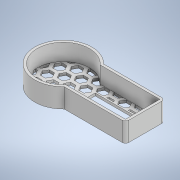
# Autodesk Inventor part: badge
Saved by Autodesk Inventor 2022 (Build 260153000, 153)
## iProperties
Created: 2019-12-22
Part Number: badge
Material: Generic
Document SubType Name: Modeling
Designer: user
Density: 1 g/cm^3
Appearance: Default
Author: user
## iProperties of the stored document _3DPrint.ipt
Created: 2019-12-23
Part Number: _3DPrint
Material: Generic
Document SubType Name: Modeling
Designer: user
Density: 1 g/cm^3
Appearance: Default
Author: user
Autodesk Inventor part; units mm, degrees
(part 1 of 2)
ref_plane "YZ Plane" through (0, 0, 0) normal (1, 0, 0) x (0, 1, 0)
ref_plane "XZ Plane" through (0, 0, 0) normal (0, 1, 0) x (-1, 0, 0)
ref_plane "XY Plane" through (0, 0, 0) normal (0, 0, 1) x (1, 0, 0)
sketch "Sketch1" plane through (0, 0, 0) normal (0, 1, 0) x (-1, 0, 0)
  line L0 (10.663939, 24.188791) -> (-74.736061, 24.188791)
  line L1 (-74.736061, -33.711209) -> (10.663939, -33.711209)
  line L2 (12.663939, 15.288573) -> (20.571727, 5.864438)
  line L3 (21.039638, 4.578863) -> (21.039638, -14.141384)
  line L4 (20.571727, -15.42696) -> (12.663939, -24.851094)
  circle A0 centre (-13.836061, -4.761209) radius 17
  line L5 (-62.621724, 4.988791) -> (-62.621724, -14.511209)
  line L6 (-60.621724, -16.511209) -> (-26.121724, -16.511209)
  line L7 (-26.121724, 6.988791) -> (-60.621724, 6.988791)
  arc A1 (-62.621724, -14.511209) -> (-60.621724, -16.511209) centre (-60.621724, -14.511209) ccw
  arc A2 (-60.621724, 6.988791) -> (-62.621724, 4.988791) centre (-60.621724, 4.988791) ccw
  line L8 (-28.586061, -0.511209) -> (-55.121724, -0.511209)
  line L9 (-55.121724, -0.511209) -> (-55.121724, -9.011209)
  line L10 (-55.121724, -9.011209) -> (-28.586061, -9.011209)
  line L11 (-28.586061, -9.011209) -> (-28.586061, -0.511209)
  line L12 (-76.736061, 6.188791) -> (-76.736061, 22.188791)
  line L13 (-76.736061, -15.711209) -> (-76.736061, -31.711209)
  line L14 (9.163939, 22.688791) -> (-73.236061, 22.688791)
  line L15 (-73.236061, -32.211209) -> (9.163939, -32.211209)
  line L16 (11.163939, -30.211209) -> (11.163939, 20.688791)
  line L17 (-75.236061, 20.688791) -> (-75.236061, 4.86332)
  line L18 (-75.236061, -30.211209) -> (-75.236061, -14.385738)
  line L19 (12.663939, 22.188791) -> (12.663939, 15.288573)
  line L20 (12.663939, -24.851094) -> (12.663939, -31.711209)
  arc A3 (-76.736061, -31.711209) -> (-74.736061, -33.711209) centre (-74.736061, -31.711209) ccw
  arc A4 (-75.236061, -30.211209) -> (-73.236061, -32.211209) centre (-73.236061, -30.211209) ccw
  arc A5 (-73.236061, 22.688791) -> (-75.236061, 20.688791) centre (-73.236061, 20.688791) ccw
  arc A6 (-74.736061, 24.188791) -> (-76.736061, 22.188791) centre (-74.736061, 22.188791) ccw
  arc A7 (12.663939, 22.188791) -> (10.663939, 24.188791) centre (10.663939, 22.188791) ccw
  arc A8 (11.163939, 20.688791) -> (9.163939, 22.688791) centre (9.163939, 20.688791) ccw
  arc A9 (9.163939, -32.211209) -> (11.163939, -30.211209) centre (9.163939, -30.211209) ccw
  arc A10 (10.663939, -33.711209) -> (12.663939, -31.711209) centre (10.663939, -31.711209) ccw
  arc A11 (20.571727, -15.42696) -> (21.039638, -14.141384) centre (19.039638, -14.141384) ccw
  arc A12 (21.039638, 4.578863) -> (20.571727, 5.864438) centre (19.039638, 4.578863) ccw
  arc A13 (-76.736061, -15.711209) -> (-76.736061, 6.188791) centre (-85.076375, -4.761209) ccw
  circle A14 centre (16.664118, 5.166112) radius 1.75
  circle A15 centre (16.664118, -14.728633) radius 1.75
  line L21 (12.663939, 15.288573) -> (12.663939, -24.851094)
  line L22 (18.425716, 0.463151) -> (18.425716, -9.93338)
  line L23 (14.925716, 0.440313) -> (14.925716, -10.09463)
  arc A16 (14.925716, -10.09463) -> (18.425716, -9.93338) centre (16.664118, -9.762269) ccw
  arc A17 (18.425716, 0.463151) -> (14.925716, 0.440313) centre (16.67736, 0.199747) ccw
  point P0 (0, 0)
  point P1 (12.663939, 24.188791)
  point P2 (-76.736061, -33.711209)
  point P3 (-76.736061, 24.188791)
  point P4 (12.663939, -33.711209)
  point P5 (21.039638, -14.869325)
  point P6 (-62.621724, -16.511209)
  dimension "d19" = 18
  dimension "d20" = 34
  dimension "d26" = 2
  dimension "d28" = 7.5
  dimension "d32" = 7.5
  dimension "d33" = 7.5
  dimension "d36" = 1.5
  dimension "d37" = 1.5
  dimension "d40" = 1.5
  dimension "d41" = 2
  dimension "d84" = 54.9
  dimension "d89" = 18
  dimension "d104" = 86.4
  dimension "d110" = 13.76457
  dimension "d116" = 1.5
  dimension "d122" = 3.5
  dimension "d123" = 3.5
  dimension "d124" = 3.44228
  dimension "d125" = 3.44228
  dimension "d155" = 25
  dimension "d163" = 15.7
  dimension "d164" = 15.7
  dimension "d165" = 27.45
  dimension "d166" = 27.45
  dimension "d167" = 8.5
  dimension "d171" = 26.53566
  dimension "d173" = 39.75
  dimension "d213" = 4.00018
  dimension "d214" = 4.00018
  dimension "d219" = 140
  dimension "d221" = 140
  dimension "d246" = 4.96636
  dimension "d247" = 4.96636
  dimension "d248" = 13.5
  dimension "d249" = 1.5
  dimension "d250" = 1.5
  dimension "d251" = 4.00018
  dimension "d262" = 3.5
  dimension "d263" = 2.61392
  constraints: 48 end point, 34 point on circle, 24 tangent, 18 centre point, 13 point on line, 10 equal radius, 6 vertical, 5 parallel, 3 horizontal, 3 perpendicular, 2 collinear
  measures "d19" distance of point (-76.736, 24.189) L12.start
  measures "d20" diameter of A0
  measures "d26" radius of A1
  measures "d28" distance between parallel lines of L6 L10
  measures "d32" distance between parallel lines of L8 L7
  measures "d33" distance between parallel lines of L5 L9
  measures "d36" distance between parallel lines of L0 L14
  measures "d37" distance between parallel lines of L1 L15
  measures "d40" distance between parallel lines of L13 L18
  measures "d41" radius of A3
  measures "d84" distance between parallel lines of L15 L14
  measures "d89" distance of L13.start point (-76.736, -33.711)
  measures "d104" distance between parallel lines of L17 L16
  measures "d110" radius of A13
  measures "d116" distance between parallel lines of L17 L12
  measures "d122" diameter of A15
  measures "d123" diameter of A14
  measures "d124" distance from line of L4 A15.centre
  measures "d125" distance from line of L2 A14.centre
  measures "d155" distance from line of L16 A0.centre
  measures "d163" distance between parallel lines of L15 L6
  measures "d164" distance between parallel lines of L14 L7
  measures "d165" distance from line of L15 A0.centre
  measures "d166" distance from line of L14 A0.centre
  measures "d167" distance between parallel lines of L8 L10
  measures "d171" distance between parallel lines of L9 L11
  measures "d173" distance between parallel lines of L16 L11
  measures "d213" distance from line of L21 A14.centre
  measures "d214" distance from line of L21 A15.centre
  measures "d219" angle of L19 L2
  measures "d221" angle of L20 L4
  measures "d246" distance of A17.centre A14.centre
  measures "d247" distance of A15.centre A16.centre
  measures "d249" distance between parallel lines of L16 L19
  measures "d250" distance between parallel lines of L16 L20
  measures "d251" distance from line of L21 A16.centre
  measures "d262" distance between parallel lines of L23 L22
  measures "d263" distance from line of L3 L22.end
sketch "Sketch1 outline for TokenBuffer" plane through (0, 0, 0) normal (0, 1, 0) x (-1, 0, 0)
  line L0 (-26.121724, 6.988791) -> (-60.621724, 6.988791)
  arc A0 (-26.121724, -16.511209) -> (-26.121724, 6.988791) centre (-13.836061, -4.761209) ccw
  arc A1 (-60.621724, 6.988791) -> (-62.621724, 4.988791) centre (-60.621724, 4.988791) ccw
  line L1 (-60.621724, -16.511209) -> (-26.121724, -16.511209)
  line L2 (-62.621724, 4.988791) -> (-62.621724, -14.511209)
  arc A2 (-62.621724, -14.511209) -> (-60.621724, -16.511209) centre (-60.621724, -14.511209) ccw
  line L3 (-55.121724, -0.511209) -> (-28.586061, -0.511209)
  line L4 (-55.121724, -9.011209) -> (-55.121724, -0.511209)
  line L5 (-28.586061, -9.011209) -> (-55.121724, -9.011209)
  line L6 (-28.586061, -0.511209) -> (-28.586061, -9.011209)
extrude "TokenBuffer" add sketch "Sketch1 outline for TokenBuffer" against normal blind 10
sketch "Sketch4" plane through (0, 0, 0) normal (0, 1, 0) x (1, 0, 0)
  arc A0 (26.121724, 16.511209) -> (26.121724, -6.988791) centre (13.836061, 4.761209) ccw
  circle A1 centre (13.836061, 4.761209) radius 15.5
  line L0 (25.463077, -5.488791) -> (61.121724, -5.488791)
  line L1 (61.121724, -5.488791) -> (61.121724, 15.011209)
  line L2 (61.121724, 15.011209) -> (25.463077, 15.011209)
  line L3 (25.463077, 15.011209) -> (25.463077, -5.488791)
  line L4 (60.621724, -6.988791) -> (26.121724, -6.988791)
  line L5 (26.121724, 16.511209) -> (60.621724, 16.511209)
  line L6 (62.621724, 14.511209) -> (62.621724, -4.988791)
  point P0 (0, 0)
  point P1 (25.463077, 15.011209)
  point P2 (25.463077, 15.011209)
  dimension "d56" = 1.5
  dimension "d57" = 1.5
  dimension "d58" = 1.5
  dimension "d59" = 1.5
  constraints: 8 end point, 2 parallel, 1 coincident, 1 horizontal, 1 perpendicular, 3 other
  measures "d57" distance between parallel lines of L4 L0
  measures "d58" distance between parallel lines of L5 L2
  measures "d59" distance between parallel lines of L6 L1
sketch "Sketch4 outline for TokenCut" plane through (0, 0, 0) normal (0, 1, 0) x (1, 0, 0)
  arc A0 (25.463077, 15.011209) -> (25.463077, -5.488791) centre (13.836061, 4.761209) ccw
  line L0 (61.121724, 15.011209) -> (25.463077, 15.011209)
  line L1 (61.121724, -5.488791) -> (61.121724, 15.011209)
  line L2 (25.463077, -5.488791) -> (61.121724, -5.488791)
extrude "TokenCut" cut sketch "Sketch4 outline for TokenCut" against normal blind 8.5
sketch "Sketch12" plane through (0, 0, 0) normal (0, 1, 0) x (1, 0, 0)
  arc A0 (25.463077, 15.011209) -> (25.463077, -5.488791) centre (13.836061, 4.761209) ccw
  circle A1 centre (13.836061, 4.761209) radius 15.5
  line L0 (60.621724, -6.988791) -> (26.121724, -6.988791)
  line L1 (26.121724, -6.988791) -> (60.621724, -6.988791)
  line L2 (62.621724, 14.511209) -> (62.621724, -4.988791)
  arc A2 (60.621724, -6.988791) -> (62.621724, -4.988791) centre (60.621724, -4.988791) ccw
  line L3 (61.121724, -5.488791) -> (25.463077, -5.488791)
  line L4 (25.463077, -5.488791) -> (61.121724, -5.488791)
  line L5 (61.121724, 15.011209) -> (61.121724, -5.488791)
  line L6 (61.121724, -5.488791) -> (61.121724, 15.011209)
  line L7 (25.463077, 15.011209) -> (61.121724, 15.011209)
  line L8 (61.121724, 15.011209) -> (25.463077, 15.011209)
  line L9 (62.621724, -4.988791) -> (63.064996, 19.511209)
  line L10 (62.621724, 14.511209) -> (62.621724, -4.988791)
  line L11 (62.621724, -4.988791) -> (62.621724, 14.511209)
  line L12 (26.121724, 16.511209) -> (60.621724, 16.511209)
  arc A3 (62.621724, 14.511209) -> (60.621724, 16.511209) centre (60.621724, 14.511209) ccw
  line L13 (60.621724, 16.511209) -> (26.121724, 16.511209)
  circle A4 centre (13.836061, 4.761209) radius 17
  point P0 (0, 0)
  point P1 (26.121724, 16.511209)
  dimension "d152" = 34
  constraints: 14 end point, 4 centre point, 4 point on circle, 2 coincident, 2 horizontal, 2 perpendicular, 1 collinear, 1 tangent
  measures "d152" diameter of A4
sketch "Sketch12 outline for TokenAddition" plane through (0, 0, 0) normal (0, 1, 0) x (1, 0, 0)
  arc A0 (26.121724, 16.511209) -> (26.121724, -6.988791) centre (13.836061, 4.761209) ccw
  line L0 (60.621724, 16.511209) -> (26.121724, 16.511209)
  line L1 (26.121724, -6.988791) -> (60.621724, -6.988791)
  arc A1 (62.621724, 14.511209) -> (60.621724, 16.511209) centre (60.621724, 14.511209) ccw
  arc A2 (60.621724, -6.988791) -> (62.621724, -4.988791) centre (60.621724, -4.988791) ccw
  line L2 (62.621724, -4.988791) -> (62.621724, 14.511209)
  line L3 (25.463077, 15.011209) -> (61.121724, 15.011209)
  arc A3 (25.463077, -5.488791) -> (25.463077, 15.011209) centre (13.836061, 4.761209) cw
  line L4 (61.121724, -5.488791) -> (25.463077, -5.488791)
  line L5 (61.121724, 15.011209) -> (61.121724, -5.488791)
extrude "TokenAddition" add sketch "Sketch12 outline for TokenAddition" along normal blind 1.5
sketch "Sketch23" plane through (0, -10, 0) normal (0, -1, 0) x (1, 0, 0)
  line L0 (7.80058, -8.259557) -> (9.35908, -5.560156)
  line L1 (9.35908, -5.560156) -> (12.47608, -5.560156)
  line L2 (12.47608, -5.560156) -> (14.03458, -8.259557)
  line L3 (14.03458, -8.259557) -> (12.47608, -10.958958)
  line L4 (12.47608, -10.958958) -> (9.35908, -10.958958)
  line L5 (9.35908, -10.958958) -> (7.80058, -8.259557)
  line L6 (6.645879, -8.259557) -> (8.781729, -4.560156)
  line L7 (8.781729, -4.560156) -> (13.05343, -4.560156)
  line L8 (13.05343, -4.560156) -> (15.18928, -8.259557)
  line L9 (15.18928, -8.259557) -> (13.05343, -11.958958)
  line L10 (13.05343, -11.958958) -> (8.781729, -11.958958)
  line L11 (8.781729, -11.958958) -> (6.645879, -8.259557)
  line L12 (18.883631, -1.860755) -> (15.766631, -1.860755)
  line L13 (15.766631, -1.860755) -> (14.208131, -4.560156)
  line L14 (14.208131, -4.560156) -> (15.766631, -7.259557)
  line L15 (15.766631, -7.259557) -> (18.883631, -7.259557)
  line L16 (18.883631, -7.259557) -> (20.442131, -4.560156)
  line L17 (20.442131, -4.560156) -> (18.883631, -1.860755)
  line L18 (19.460981, -0.860755) -> (15.18928, -0.860755)
  line L19 (15.18928, -0.860755) -> (13.05343, -4.560156)
  line L20 (15.18928, -8.259557) -> (19.460981, -8.259557)
  line L21 (19.460981, -8.259557) -> (21.596831, -4.560156)
  line L22 (21.596831, -4.560156) -> (19.460981, -0.860755)
  line L23 (31.698732, 5.538047) -> (28.581732, 5.538047)
  line L24 (28.581732, 5.538047) -> (27.023232, 2.838646)
  line L25 (27.023232, 2.838646) -> (28.581732, 0.139245)
  line L26 (28.581732, 0.139245) -> (31.698732, 0.139245)
  line L27 (31.698732, 0.139245) -> (33.257232, 2.838646)
  line L28 (33.257232, 2.838646) -> (31.698732, 5.538047)
  line L29 (32.276082, 6.538047) -> (28.004382, 6.538047)
  line L30 (28.004382, 6.538047) -> (25.868532, 2.838646)
  line L31 (25.868532, 2.838646) -> (28.004382, -0.860755)
  line L32 (28.004382, -0.860755) -> (32.276082, -0.860755)
  line L33 (32.276082, -0.860755) -> (34.411933, 2.838646)
  line L34 (34.411933, 2.838646) -> (32.276082, 6.538047)
  line L35 (20.615681, -0.860755) -> (22.174181, 1.838646)
  line L36 (22.174181, 1.838646) -> (25.291181, 1.838646)
  line L37 (25.291181, 1.838646) -> (26.849681, -0.860755)
  line L38 (26.849681, -0.860755) -> (25.291181, -3.560156)
  line L39 (25.291181, -3.560156) -> (22.174181, -3.560156)
  line L40 (22.174181, -3.560156) -> (20.615681, -0.860755)
  line L41 (19.460981, -0.860755) -> (21.596831, 2.838646)
  line L42 (21.596831, 2.838646) -> (25.868532, 2.838646)
  line L43 (28.004382, -0.860755) -> (25.868532, -4.560156)
  line L44 (25.868532, -4.560156) -> (21.596831, -4.560156)
  line L45 (7.80058, -0.860755) -> (9.35908, -3.560156)
  line L46 (9.35908, -3.560156) -> (12.47608, -3.560156)
  line L47 (12.47608, -3.560156) -> (14.03458, -0.860755)
  line L48 (14.03458, -0.860755) -> (12.47608, 1.838646)
  line L49 (12.47608, 1.838646) -> (9.35908, 1.838646)
  line L50 (9.35908, 1.838646) -> (7.80058, -0.860755)
  line L51 (6.645879, -0.860755) -> (8.781729, -4.560156)
  line L52 (13.05343, -4.560156) -> (15.18928, -0.860755)
  line L53 (15.18928, -0.860755) -> (13.05343, 2.838646)
  line L54 (13.05343, 2.838646) -> (8.781729, 2.838646)
  line L55 (8.781729, 2.838646) -> (6.645879, -0.860755)
  line L56 (8.781729, 10.237449) -> (13.05343, 10.237449)
  line L57 (15.18928, 6.538047) -> (13.05343, 10.237449)
  line L58 (7.80058, 6.538047) -> (9.35908, 9.237449)
  line L59 (9.35908, 9.237449) -> (12.47608, 9.237449)
  line L60 (12.47608, 3.838646) -> (9.35908, 3.838646)
  line L61 (9.35908, 3.838646) -> (7.80058, 6.538047)
  line L62 (6.645879, 6.538047) -> (8.781729, 10.237449)
  line L63 (8.781729, 2.838646) -> (6.645879, 6.538047)
  line L64 (12.47608, 9.237449) -> (14.03458, 6.538047)
  line L65 (15.18928, 6.538047) -> (13.05343, 2.838646)
  line L66 (14.03458, 6.538047) -> (12.47608, 3.838646)
  line L67 (6.645879, -0.860755) -> (8.781729, 2.838646)
  line L68 (6.645879, 6.538047) -> (2.374179, 6.538047)
  line L69 (6.068529, 5.538047) -> (2.951529, 5.538047)
  line L70 (2.951529, 5.538047) -> (1.393029, 2.838646)
  line L71 (2.374179, 6.538047) -> (0.238328, 2.838646)
  line L72 (2.374179, -0.860755) -> (0.238328, 2.838646)
  line L73 (1.393029, 2.838646) -> (2.951529, 0.139245)
  line L74 (2.951529, 0.139245) -> (6.068529, 0.139245)
  line L75 (2.374179, -0.860755) -> (6.645879, -0.860755)
  line L76 (6.068529, 0.139245) -> (7.627029, 2.838646)
  line L77 (7.627029, 2.838646) -> (6.068529, 5.538047)
  line L78 (8.781729, -4.560156) -> (6.645879, -0.860755)
  line L79 (8.781729, -4.560156) -> (6.645879, -8.259557)
  line L80 (1.393029, -4.560156) -> (2.951529, -1.860755)
  line L81 (2.374179, -0.860755) -> (0.238328, -4.560156)
  line L82 (2.374179, -8.259557) -> (0.238328, -4.560156)
  line L83 (6.068529, -7.259557) -> (2.951529, -7.259557)
  line L84 (6.645879, -8.259557) -> (2.374179, -8.259557)
  line L85 (2.951529, -7.259557) -> (1.393029, -4.560156)
  line L86 (6.068529, -1.860755) -> (7.627029, -4.560156)
  line L87 (2.951529, -1.860755) -> (6.068529, -1.860755)
  line L88 (7.627029, -4.560156) -> (6.068529, -7.259557)
  line L89 (6.645879, -8.259557) -> (8.781729, -11.958958)
  line L90 (6.645879, -15.65836) -> (8.781729, -11.958958)
  line L91 (2.374179, -15.65836) -> (6.645879, -15.65836)
  line L92 (2.951529, -14.65836) -> (6.068529, -14.65836)
  line L93 (6.068529, -14.65836) -> (7.627029, -11.958958)
  line L94 (7.627029, -11.958958) -> (6.068529, -9.259557)
  line L95 (6.068529, -9.259557) -> (2.951529, -9.259557)
  line L96 (2.374179, -8.259557) -> (0.238328, -11.958958)
  line L97 (2.951529, -9.259557) -> (1.393029, -11.958958)
  line L98 (1.393029, -11.958958) -> (2.951529, -14.65836)
  line L99 (2.374179, -15.65836) -> (0.238328, -11.958958)
  line L100 (8.781729, -11.958958) -> (13.05343, -11.958958)
  line L101 (13.05343, -11.958958) -> (15.18928, -15.65836)
  line L102 (9.35908, -18.357761) -> (7.80058, -15.65836)
  line L103 (8.781729, -19.357761) -> (6.645879, -15.65836)
  line L104 (7.80058, -15.65836) -> (9.35908, -12.958958)
  line L105 (9.35908, -12.958958) -> (12.47608, -12.958958)
  line L106 (12.47608, -12.958958) -> (14.03458, -15.65836)
  line L107 (14.03458, -15.65836) -> (12.47608, -18.357761)
  line L108 (15.18928, -15.65836) -> (13.05343, -19.357761)
  line L109 (12.47608, -18.357761) -> (9.35908, -18.357761)
  line L110 (8.781729, -19.357761) -> (13.05343, -19.357761)
  line L111 (21.596831, 2.838646) -> (19.460981, -0.860755)
  line L112 (15.18928, -0.860755) -> (19.460981, -0.860755)
  line L113 (18.883631, 5.538047) -> (20.442131, 2.838646)
  line L114 (20.442131, 2.838646) -> (18.883631, 0.139245)
  line L115 (14.208131, 2.838646) -> (15.766631, 5.538047)
  line L116 (15.766631, 5.538047) -> (18.883631, 5.538047)
  line L117 (19.460981, 6.538047) -> (21.596831, 2.838646)
  line L118 (13.05343, 2.838646) -> (15.18928, 6.538047)
  line L119 (15.18928, 6.538047) -> (19.460981, 6.538047)
  line L120 (18.883631, 0.139245) -> (15.766631, 0.139245)
  line L121 (15.766631, 0.139245) -> (14.208131, 2.838646)
  line L122 (19.460981, -8.259557) -> (15.18928, -8.259557)
  line L123 (18.883631, -9.259557) -> (15.766631, -9.259557)
  line L124 (15.18928, -8.259557) -> (13.05343, -11.958958)
  line L125 (15.766631, -9.259557) -> (14.208131, -11.958958)
  line L126 (14.208131, -11.958958) -> (15.766631, -14.65836)
  line L127 (15.766631, -14.65836) -> (18.883631, -14.65836)
  line L128 (15.18928, -15.65836) -> (19.460981, -15.65836)
  line L129 (18.883631, -14.65836) -> (20.442131, -11.958958)
  line L130 (21.596831, -11.958958) -> (19.460981, -15.65836)
  line L131 (20.442131, -11.958958) -> (18.883631, -9.259557)
  line L132 (21.596831, -11.958958) -> (19.460981, -8.259557)
  line L133 (21.596831, -4.560156) -> (25.868532, -4.560156)
  line L134 (21.596831, -4.560156) -> (19.460981, -8.259557)
  line L135 (25.868532, -4.560156) -> (28.004382, -8.259557)
  line L136 (25.291181, -5.560156) -> (26.849681, -8.259557)
  line L137 (22.174181, -5.560156) -> (25.291181, -5.560156)
  line L138 (22.174181, -10.958958) -> (20.615681, -8.259557)
  line L139 (20.615681, -8.259557) -> (22.174181, -5.560156)
  line L140 (25.291181, -10.958958) -> (22.174181, -10.958958)
  line L141 (21.596831, -11.958958) -> (25.868532, -11.958958)
  line L142 (28.004382, -8.259557) -> (25.868532, -11.958958)
  line L143 (26.849681, -8.259557) -> (25.291181, -10.958958)
  line L144 (33.430783, 6.538047) -> (34.989283, 9.237449)
  line L145 (34.989283, 9.237449) -> (38.106283, 9.237449)
  line L146 (38.106283, 9.237449) -> (39.664783, 6.538047)
  line L147 (39.664783, 6.538047) -> (38.106283, 3.838646)
  line L148 (38.106283, 3.838646) -> (34.989283, 3.838646)
  line L149 (34.989283, 3.838646) -> (33.430783, 6.538047)
  line L150 (38.683633, 10.237449) -> (40.819483, 6.538047)
  line L151 (40.819483, 6.538047) -> (38.683633, 2.838646)
  line L152 (34.411933, 10.237449) -> (38.683633, 10.237449)
  line L153 (38.683633, 2.838646) -> (34.411933, 2.838646)
  line L154 (32.276082, 6.538047) -> (34.411933, 10.237449)
  line L155 (25.868532, 2.838646) -> (28.004382, 6.538047)
  line L156 (25.868532, 2.838646) -> (21.596831, 2.838646)
  line L157 (28.004382, 6.538047) -> (25.868532, 10.237449)
  line L158 (21.596831, 10.237449) -> (25.868532, 10.237449)
  line L159 (26.849681, 6.538047) -> (25.291181, 9.237449)
  line L160 (25.291181, 9.237449) -> (22.174181, 9.237449)
  line L161 (21.596831, 10.237449) -> (19.460981, 6.538047)
  line L162 (22.174181, 9.237449) -> (20.615681, 6.538047)
  line L163 (20.615681, 6.538047) -> (22.174181, 3.838646)
  line L164 (22.174181, 3.838646) -> (25.291181, 3.838646)
  line L165 (25.291181, 3.838646) -> (26.849681, 6.538047)
  line L166 (19.460981, 13.93685) -> (15.18928, 13.93685)
  line L167 (19.460981, 13.93685) -> (21.596831, 10.237449)
  line L168 (15.18928, 13.93685) -> (13.05343, 10.237449)
  line L169 (15.18928, 6.538047) -> (13.05343, 10.237449)
  line L170 (15.766631, 12.93685) -> (14.208131, 10.237449)
  line L171 (14.208131, 10.237449) -> (15.766631, 7.538047)
  line L172 (15.766631, 7.538047) -> (18.883631, 7.538047)
  line L173 (18.883631, 7.538047) -> (20.442131, 10.237449)
  line L174 (19.460981, 6.538047) -> (21.596831, 10.237449)
  line L175 (20.442131, 10.237449) -> (18.883631, 12.93685)
  line L176 (18.883631, 12.93685) -> (15.766631, 12.93685)
  line L177 (13.05343, 17.636251) -> (8.781729, 17.636251)
  line L178 (6.645879, 13.93685) -> (8.781729, 10.237449)
  line L179 (7.80058, 13.93685) -> (9.35908, 11.237449)
  line L180 (9.35908, 11.237449) -> (12.47608, 11.237449)
  line L181 (15.18928, 13.93685) -> (13.05343, 10.237449)
  line L182 (12.47608, 11.237449) -> (14.03458, 13.93685)
  line L183 (14.03458, 13.93685) -> (12.47608, 16.636251)
  line L184 (15.18928, 13.93685) -> (13.05343, 17.636251)
  line L185 (12.47608, 16.636251) -> (9.35908, 16.636251)
  line L186 (8.781729, 17.636251) -> (6.645879, 13.93685)
  line L187 (9.35908, 16.636251) -> (7.80058, 13.93685)
  line L188 (8.781729, 10.237449) -> (6.645879, 13.93685)
  line L189 (8.781729, 10.237449) -> (6.645879, 6.538047)
  line L190 (1.393029, 10.237449) -> (2.951529, 12.93685)
  line L191 (2.374179, 13.93685) -> (0.238328, 10.237449)
  line L192 (2.374179, 6.538047) -> (0.238328, 10.237449)
  line L193 (6.068529, 7.538047) -> (2.951529, 7.538047)
  line L194 (2.951529, 7.538047) -> (1.393029, 10.237449)
  line L195 (6.068529, 12.93685) -> (7.627029, 10.237449)
  line L196 (2.951529, 12.93685) -> (6.068529, 12.93685)
  line L197 (2.374179, 13.93685) -> (6.645879, 13.93685)
  line L198 (7.627029, 10.237449) -> (6.068529, 7.538047)
  line L199 (-6.169222, -0.860755) -> (-4.033372, 2.838646)
  line L200 (0.238328, 2.838646) -> (-4.033372, 2.838646)
  line L201 (2.374179, -0.860755) -> (0.238328, 2.838646)
  line L202 (1.219478, -0.860755) -> (-0.339022, 1.838646)
  line L203 (-0.339022, 1.838646) -> (-3.456022, 1.838646)
  line L204 (-3.456022, 1.838646) -> (-5.014522, -0.860755)
  line L205 (-6.169222, -0.860755) -> (-4.033372, -4.560156)
  line L206 (-5.014522, -0.860755) -> (-3.456022, -3.560156)
  line L207 (-4.033372, -4.560156) -> (0.238328, -4.560156)
  line L208 (-3.456022, -3.560156) -> (-0.339022, -3.560156)
  line L209 (-0.339022, -3.560156) -> (1.219478, -0.860755)
  line L210 (-4.033372, -4.560156) -> (0.238328, -4.560156)
  line L211 (0.238328, -4.560156) -> (2.374179, -8.259557)
  line L212 (-3.456022, -10.958958) -> (-5.014522, -8.259557)
  line L213 (-4.033372, -11.958958) -> (-6.169222, -8.259557)
  line L214 (-5.014522, -8.259557) -> (-3.456022, -5.560156)
  line L215 (-6.169222, -8.259557) -> (-4.033372, -4.560156)
  line L216 (-3.456022, -5.560156) -> (-0.339022, -5.560156)
  line L217 (-0.339022, -5.560156) -> (1.219478, -8.259557)
  line L218 (1.219478, -8.259557) -> (-0.339022, -10.958958)
  line L219 (-0.339022, -10.958958) -> (-3.456022, -10.958958)
  line L220 (-4.033372, -11.958958) -> (0.238328, -11.958958)
  line L221 (19.460981, -15.65836) -> (21.596831, -19.357761)
  line L222 (19.460981, -23.057162) -> (21.596831, -19.357761)
  line L223 (18.883631, -22.057162) -> (20.442131, -19.357761)
  line L224 (20.442131, -19.357761) -> (18.883631, -16.65836)
  line L225 (19.460981, -15.65836) -> (15.18928, -15.65836)
  line L226 (18.883631, -16.65836) -> (15.766631, -16.65836)
  line L227 (15.766631, -16.65836) -> (14.208131, -19.357761)
  line L228 (14.208131, -19.357761) -> (15.766631, -22.057162)
  line L229 (15.18928, -23.057162) -> (13.05343, -19.357761)
  line L230 (15.766631, -22.057162) -> (18.883631, -22.057162)
  line L231 (15.18928, -23.057162) -> (19.460981, -23.057162)
  line L232 (8.781729, -19.357761) -> (6.645879, -23.057162)
  line L233 (6.645879, -23.057162) -> (2.374179, -23.057162)
  line L234 (2.951529, -16.65836) -> (6.068529, -16.65836)
  line L235 (6.068529, -16.65836) -> (7.627029, -19.357761)
  line L236 (6.645879, -15.65836) -> (8.781729, -19.357761)
  line L237 (7.627029, -19.357761) -> (6.068529, -22.057162)
  line L238 (6.068529, -22.057162) -> (2.951529, -22.057162)
  line L239 (2.951529, -22.057162) -> (1.393029, -19.357761)
  line L240 (2.374179, -23.057162) -> (0.238328, -19.357761)
  line L241 (1.393029, -19.357761) -> (2.951529, -16.65836)
  line L242 (2.374179, -15.65836) -> (0.238328, -19.357761)
  arc A0 (26.238399, 7.066705) -> (26.121724, -16.511209) centre (13.932065, -4.661643) ccw
  arc A1 (62.474431, 5.742101) -> (60.621724, 6.988791) centre (60.621724, 4.988791) ccw
  line L243 (26.238399, 7.066705) -> (60.621724, 7.066705)
  line L244 (62.621724, -14.511209) -> (62.621724, 4.988791)
  line L245 (62.738399, 5.430757) -> (62.738399, -14.511209)
  arc A2 (62.474431, 5.742101) -> (60.621724, 6.988791) centre (60.621724, 4.988791) ccw
  arc A3 (60.621724, -16.511209) -> (62.621724, -14.511209) centre (60.621724, -14.511209) ccw
  arc A4 (60.621724, -16.511209) -> (62.621724, -14.511209) centre (60.621724, -14.511209) ccw
  line L246 (26.121724, -16.511209) -> (60.621724, -16.511209)
  line L247 (60.621724, -16.511209) -> (26.121724, -16.511209)
  line L248 (61.238399, 5.566705) -> (61.238399, 4.11735)
  line L249 (61.238399, 4.11735) -> (61.238399, -14.933295)
  line L250 (61.238399, 5.566705) -> (26.288877, 5.566705)
  line L251 (61.238399, -14.933295) -> (25.463077, -14.933295)
  arc A5 (25.463077, 5.488791) -> (25.463077, -15.011209) centre (13.836061, -4.761209) ccw
  arc A6 (25.827358, 5.488791) -> (25.463077, -15.011209) centre (13.936454, -4.553147) ccw
  line L252 (27.176069, 7.736642) -> (26.727358, 6.988791)
  line L253 (25.827358, 5.566705) -> (26.288877, 5.566705)
  line L254 (25.827358, 5.488791) -> (31.511345, 5.488791)
  line L255 (28.004382, -15.65836) -> (25.868532, -19.357761)
  line L256 (28.004382, -15.65836) -> (25.868532, -11.958958)
  line L257 (25.868532, -19.357761) -> (21.596831, -19.357761)
  line L258 (25.291181, -18.357761) -> (22.174181, -18.357761)
  line L259 (26.849681, -15.65836) -> (25.291181, -18.357761)
  line L260 (22.174181, -12.958958) -> (25.291181, -12.958958)
  line L261 (25.291181, -12.958958) -> (26.849681, -15.65836)
  line L262 (21.596831, -11.958958) -> (25.868532, -11.958958)
  line L263 (20.615681, -15.65836) -> (22.174181, -12.958958)
  line L264 (21.596831, -19.357761) -> (19.460981, -15.65836)
  line L265 (22.174181, -18.357761) -> (20.615681, -15.65836)
  line L266 (28.004382, -8.259557) -> (32.276082, -8.259557)
  line L267 (28.004382, -8.259557) -> (25.868532, -11.958958)
  line L268 (32.276082, -8.259557) -> (34.411933, -11.958958)
  line L269 (31.698732, -9.259557) -> (28.581732, -9.259557)
  line L270 (33.257232, -11.958958) -> (31.698732, -9.259557)
  line L271 (32.276082, -15.65836) -> (34.411933, -11.958958)
  line L272 (31.698732, -14.65836) -> (33.257232, -11.958958)
  line L273 (28.581732, -14.65836) -> (31.698732, -14.65836)
  line L274 (28.004382, -15.65836) -> (32.276082, -15.65836)
  line L275 (27.023232, -11.958958) -> (28.581732, -14.65836)
  line L276 (28.581732, -9.259557) -> (27.023232, -11.958958)
  line L277 (28.004382, -8.259557) -> (25.868532, -11.958958)
  line L278 (55.121724, -0.511209) -> (55.121724, -9.011209)
  line L279 (55.238399, -9.011209) -> (55.238399, -0.511209)
  line L280 (28.586061, -0.511209) -> (55.121724, -0.511209)
  line L281 (55.121724, -0.433295) -> (28.586061, -0.433295)
  line L282 (28.586061, -9.011209) -> (28.586061, -0.511209)
  line L283 (28.702737, -0.511209) -> (28.702737, -9.011209)
  line L284 (55.121724, -9.011209) -> (28.586061, -9.011209)
  line L285 (28.586061, -8.933295) -> (55.121724, -8.933295)
  line L286 (56.238399, -9.933295) -> (27.702737, -9.933295)
  line L287 (27.702737, -9.933295) -> (27.702737, 0.566705)
  line L288 (27.702737, 0.566705) -> (56.238399, 0.566705)
  line L289 (56.238399, 0.566705) -> (56.238399, -9.933295)
  line L290 (40.819483, -15.65836) -> (38.683633, -19.357761)
  line L291 (34.411933, -19.357761) -> (38.683633, -19.357761)
  line L292 (38.106283, -18.357761) -> (34.989283, -18.357761)
  line L293 (34.989283, -18.357761) -> (33.430783, -15.65836)
  line L294 (34.411933, -19.357761) -> (32.276082, -15.65836)
  line L295 (33.430783, -15.65836) -> (34.989283, -12.958958)
  line L296 (38.683633, -11.958958) -> (34.411933, -11.958958)
  line L297 (34.989283, -12.958958) -> (38.106283, -12.958958)
  line L298 (40.819483, -15.65836) -> (38.683633, -11.958958)
  line L299 (38.106283, -12.958958) -> (39.664783, -15.65836)
  line L300 (39.664783, -15.65836) -> (38.106283, -18.357761)
  line L301 (45.091184, -8.259557) -> (40.819483, -8.259557)
  line L302 (44.513834, -9.259557) -> (41.396834, -9.259557)
  line L303 (47.227034, -11.958958) -> (45.091184, -8.259557)
  line L304 (46.072334, -11.958958) -> (44.513834, -9.259557)
  line L305 (44.513834, -14.65836) -> (46.072334, -11.958958)
  line L306 (47.227034, -11.958958) -> (45.091184, -15.65836)
  line L307 (40.819483, -15.65836) -> (45.091184, -15.65836)
  line L308 (41.396834, -14.65836) -> (44.513834, -14.65836)
  line L309 (39.838334, -11.958958) -> (41.396834, -14.65836)
  line L310 (41.396834, -9.259557) -> (39.838334, -11.958958)
  line L311 (38.683633, -11.958958) -> (40.819483, -8.259557)
  line L312 (32.276082, -8.259557) -> (34.411933, -11.958958)
  line L313 (33.430783, -8.259557) -> (34.989283, -10.958958)
  line L314 (34.411933, -4.560156) -> (32.276082, -8.259557)
  line L315 (34.989283, -5.560156) -> (33.430783, -8.259557)
  line L316 (38.106283, -5.560156) -> (34.989283, -5.560156)
  line L317 (34.411933, -4.560156) -> (38.683633, -4.560156)
  line L318 (40.819483, -8.259557) -> (38.683633, -4.560156)
  line L319 (39.664783, -8.259557) -> (38.106283, -5.560156)
  line L320 (40.819483, -8.259557) -> (38.683633, -11.958958)
  line L321 (38.106283, -10.958958) -> (39.664783, -8.259557)
  line L322 (34.989283, -10.958958) -> (38.106283, -10.958958)
  line L323 (47.227034, -19.357761) -> (51.498735, -19.357761)
  line L324 (50.921385, -12.958958) -> (52.479885, -15.65836)
  line L325 (51.498735, -11.958958) -> (53.634585, -15.65836)
  line L326 (47.227034, -11.958958) -> (51.498735, -11.958958)
  line L327 (47.804385, -12.958958) -> (50.921385, -12.958958)
  line L328 (46.245885, -15.65836) -> (47.804385, -12.958958)
  line L329 (47.227034, -19.357761) -> (45.091184, -15.65836)
  line L330 (47.804385, -18.357761) -> (46.245885, -15.65836)
  line L331 (50.921385, -18.357761) -> (47.804385, -18.357761)
  line L332 (52.479885, -15.65836) -> (50.921385, -18.357761)
  line L333 (51.498735, -19.357761) -> (53.634585, -15.65836)
  line L334 (47.227034, -11.958958) -> (45.091184, -8.259557)
  line L335 (46.245885, -8.259557) -> (47.804385, -10.958958)
  line L336 (47.804385, -5.560156) -> (46.245885, -8.259557)
  line L337 (47.227034, -4.560156) -> (45.091184, -8.259557)
  line L338 (47.227034, -4.560156) -> (51.498735, -4.560156)
  line L339 (50.921385, -5.560156) -> (47.804385, -5.560156)
  line L340 (51.498735, -4.560156) -> (53.634585, -8.259557)
  line L341 (52.479885, -8.259557) -> (50.921385, -5.560156)
  line L342 (50.921385, -10.958958) -> (52.479885, -8.259557)
  line L343 (51.498735, -11.958958) -> (53.634585, -8.259557)
  line L344 (47.804385, -10.958958) -> (50.921385, -10.958958)
  line L345 (53.634585, -8.259557) -> (57.906286, -8.259557)
  line L346 (57.328935, -9.259557) -> (54.211935, -9.259557)
  line L347 (58.887435, -11.958958) -> (57.328935, -9.259557)
  line L348 (60.042136, -11.958958) -> (57.906286, -8.259557)
  line L349 (60.042136, -11.958958) -> (57.906286, -15.65836)
  line L350 (57.328935, -14.65836) -> (58.887435, -11.958958)
  line L351 (57.906286, -15.65836) -> (53.634585, -15.65836)
  line L352 (54.211935, -14.65836) -> (57.328935, -14.65836)
  line L353 (52.653435, -11.958958) -> (54.211935, -14.65836)
  line L354 (54.211935, -9.259557) -> (52.653435, -11.958958)
  line L355 (53.634585, -8.259557) -> (51.498735, -11.958958)
  line L356 (64.313836, -19.357761) -> (60.042136, -19.357761)
  line L357 (64.313836, -19.357761) -> (66.449687, -15.65836)
  line L358 (63.736486, -18.357761) -> (60.619486, -18.357761)
  line L359 (60.619486, -18.357761) -> (59.060986, -15.65836)
  line L360 (57.906286, -15.65836) -> (60.042136, -19.357761)
  line L361 (59.060986, -15.65836) -> (60.619486, -12.958958)
  line L362 (60.042136, -11.958958) -> (64.313836, -11.958958)
  line L363 (60.619486, -12.958958) -> (63.736486, -12.958958)
  line L364 (66.449687, -15.65836) -> (64.313836, -11.958958)
  line L365 (63.736486, -12.958958) -> (65.294986, -15.65836)
  line L366 (65.294986, -15.65836) -> (63.736486, -18.357761)
  line L367 (64.313836, -4.560156) -> (66.449687, -8.259557)
  line L368 (64.313836, -4.560156) -> (60.042136, -4.560156)
  line L369 (63.736486, -5.560156) -> (65.294986, -8.259557)
  line L370 (65.294986, -8.259557) -> (63.736486, -10.958958)
  line L371 (64.313836, -11.958958) -> (66.449687, -8.259557)
  line L372 (60.042136, -11.958958) -> (64.313836, -11.958958)
  line L373 (63.736486, -10.958958) -> (60.619486, -10.958958)
  line L374 (60.619486, -10.958958) -> (59.060986, -8.259557)
  line L375 (60.042136, -4.560156) -> (57.906286, -8.259557)
  line L376 (59.060986, -8.259557) -> (60.619486, -5.560156)
  line L377 (60.619486, -5.560156) -> (63.736486, -5.560156)
  line L378 (53.634585, -8.259557) -> (57.906286, -8.259557)
  line L379 (53.634585, -8.259557) -> (51.498735, -4.560156)
  line L380 (54.211935, -7.259557) -> (57.328935, -7.259557)
  line L381 (52.653435, -4.560156) -> (54.211935, -7.259557)
  line L382 (54.211935, -1.860755) -> (52.653435, -4.560156)
  line L383 (51.498735, -4.560156) -> (53.634585, -0.860755)
  line L384 (57.906286, -0.860755) -> (53.634585, -0.860755)
  line L385 (57.328935, -1.860755) -> (54.211935, -1.860755)
  line L386 (58.887435, -4.560156) -> (57.328935, -1.860755)
  line L387 (57.906286, -0.860755) -> (60.042136, -4.560156)
  line L388 (57.328935, -7.259557) -> (58.887435, -4.560156)
  line L389 (64.313836, 2.838646) -> (66.449687, -0.860755)
  line L390 (66.449687, -0.860755) -> (64.313836, -4.560156)
  line L391 (60.042136, -4.560156) -> (64.313836, -4.560156)
  line L392 (63.736486, -3.560156) -> (60.619486, -3.560156)
  line L393 (65.294986, -0.860755) -> (63.736486, -3.560156)
  line L394 (63.736486, 1.838646) -> (65.294986, -0.860755)
  line L395 (64.313836, 2.838646) -> (60.042136, 2.838646)
  line L396 (60.619486, 1.838646) -> (63.736486, 1.838646)
  line L397 (59.060986, -0.860755) -> (60.619486, 1.838646)
  line L398 (57.906286, -0.860755) -> (60.042136, 2.838646)
  line L399 (60.619486, -3.560156) -> (59.060986, -0.860755)
  line L400 (51.498735, 2.838646) -> (53.634585, 6.538047)
  line L401 (53.634585, 6.538047) -> (57.906286, 6.538047)
  line L402 (60.042136, 2.838646) -> (57.906286, 6.538047)
  line L403 (57.328935, 5.538047) -> (58.887435, 2.838646)
  line L404 (54.211935, 5.538047) -> (57.328935, 5.538047)
  line L405 (52.653435, 2.838646) -> (54.211935, 5.538047)
  line L406 (51.498735, 2.838646) -> (53.634585, -0.860755)
  line L407 (54.211935, 0.139245) -> (52.653435, 2.838646)
  line L408 (57.328935, 0.139245) -> (54.211935, 0.139245)
  line L409 (58.887435, 2.838646) -> (57.328935, 0.139245)
  line L410 (57.906286, -0.860755) -> (60.042136, 2.838646)
  line L411 (64.313836, 2.838646) -> (66.449687, 6.538047)
  line L412 (64.313836, 2.838646) -> (60.042136, 2.838646)
  line L413 (63.736486, 3.838646) -> (65.294986, 6.538047)
  line L414 (60.619486, 3.838646) -> (63.736486, 3.838646)
  line L415 (59.060986, 6.538047) -> (60.619486, 3.838646)
  line L416 (60.619486, 9.237449) -> (59.060986, 6.538047)
  line L417 (60.042136, 10.237449) -> (57.906286, 6.538047)
  line L418 (64.313836, 10.237449) -> (60.042136, 10.237449)
  line L419 (63.736486, 9.237449) -> (60.619486, 9.237449)
  line L420 (65.294986, 6.538047) -> (63.736486, 9.237449)
  line L421 (64.313836, 10.237449) -> (66.449687, 6.538047)
  line L422 (51.498735, -4.560156) -> (53.634585, -0.860755)
  line L423 (51.498735, -4.560156) -> (47.227034, -4.560156)
  line L424 (50.921385, -3.560156) -> (52.479885, -0.860755)
  line L425 (47.804385, -3.560156) -> (50.921385, -3.560156)
  line L426 (46.245885, -0.860755) -> (47.804385, -3.560156)
  line L427 (47.227034, -4.560156) -> (45.091184, -0.860755)
  line L428 (47.804385, 1.838646) -> (46.245885, -0.860755)
  line L429 (47.227034, 2.838646) -> (45.091184, -0.860755)
  line L430 (51.498735, 2.838646) -> (47.227034, 2.838646)
  line L431 (50.921385, 1.838646) -> (47.804385, 1.838646)
  line L432 (52.479885, -0.860755) -> (50.921385, 1.838646)
  line L433 (47.227034, 10.237449) -> (51.498735, 10.237449)
  line L434 (51.498735, 10.237449) -> (53.634585, 6.538047)
  line L435 (51.498735, 2.838646) -> (53.634585, 6.538047)
  line L436 (50.921385, 9.237449) -> (52.479885, 6.538047)
  line L437 (52.479885, 6.538047) -> (50.921385, 3.838646)
  line L438 (50.921385, 3.838646) -> (47.804385, 3.838646)
  line L439 (47.804385, 3.838646) -> (46.245885, 6.538047)
  line L440 (47.227034, 2.838646) -> (45.091184, 6.538047)
  line L441 (46.245885, 6.538047) -> (47.804385, 9.237449)
  line L442 (47.227034, 10.237449) -> (45.091184, 6.538047)
  line L443 (47.804385, 9.237449) -> (50.921385, 9.237449)
  line L444 (45.091184, -0.860755) -> (40.819483, -0.860755)
  line L445 (45.091184, -0.860755) -> (47.227034, 2.838646)
  line L446 (44.513834, 0.139245) -> (46.072334, 2.838646)
  line L447 (41.396834, 0.139245) -> (44.513834, 0.139245)
  line L448 (39.838334, 2.838646) -> (41.396834, 0.139245)
  line L449 (38.683633, 2.838646) -> (40.819483, -0.860755)
  line L450 (40.819483, 6.538047) -> (38.683633, 2.838646)
  line L451 (41.396834, 5.538047) -> (39.838334, 2.838646)
  line L452 (44.513834, 5.538047) -> (41.396834, 5.538047)
  line L453 (40.819483, 6.538047) -> (45.091184, 6.538047)
  line L454 (46.072334, 2.838646) -> (44.513834, 5.538047)
  line L455 (34.411933, 2.838646) -> (38.683633, 2.838646)
  line L456 (34.411933, -4.560156) -> (32.276082, -0.860755)
  line L457 (34.989283, -3.560156) -> (33.430783, -0.860755)
  line L458 (38.106283, -3.560156) -> (34.989283, -3.560156)
  line L459 (38.683633, -4.560156) -> (34.411933, -4.560156)
  line L460 (38.683633, -4.560156) -> (40.819483, -0.860755)
  line L461 (39.664783, -0.860755) -> (38.106283, -3.560156)
  line L462 (38.106283, 1.838646) -> (39.664783, -0.860755)
  line L463 (34.989283, 1.838646) -> (38.106283, 1.838646)
  line L464 (33.430783, -0.860755) -> (34.989283, 1.838646)
  line L465 (34.411933, 2.838646) -> (32.276082, -0.860755)
  point P0 (0, 0)
  point P1 (10.91758, -8.259557)
  point P2 (10.91758, -8.259557)
  point P3 (17.325131, -4.560156)
  point P4 (17.325131, -4.560156)
  point P5 (30.140232, 2.838646)
  point P6 (30.140232, 2.838646)
  point P7 (23.732681, -0.860755)
  point P8 (23.732681, -0.860755)
  point P9 (10.91758, -0.860755)
  point P10 (10.91758, -0.860755)
  point P11 (36.547783, 6.538047)
  point P12 (36.547783, 6.538047)
  point P13 (62.738399, 5.430757)
  point P14 (21.924267, 8.804584)
  point P15 (19.994829, 9.4627)
  point P16 (14.489622, 10.725006)
  point P17 (14.637371, -20.101228)
  point P18 (20.136676, -18.828698)
  point P19 (39.103978, 5.566705)
  point P20 (33.991588, 5.566705)
  point P21 (4.153922, -16.65836)
  point P22 (7.172415, -18.570347)
  point P23 (-1.594806, -5.560156)
  point P24 (-0.287781, -10.870207)
  point P25 (-0.255666, 1.69427)
  point P26 (-1.617335, -3.560156)
  point P27 (7.18363, 9.46946)
  point P28 (4.1366, 7.538047)
  point P29 (29.558487, -14.516441)
  point P30 (26.238399, -7.484622)
  point P31 (34.254928, 0.566705)
  point P32 (38.840638, 0.566705)
  point P33 (41.150039, 0.566705)
  point P34 (44.760628, 0.566705)
  point P35 (51.91908, 5.566705)
  point P36 (46.806689, 5.566705)
  point P37 (47.070029, 0.566705)
  point P38 (51.65574, 0.566705)
  point P39 (59.621791, 5.566705)
  point P40 (61.238399, 3.838646)
  point P41 (53.965141, 0.566705)
  point P42 (56.238399, 0.139245)
  point P43 (61.238399, -3.560156)
  point P44 (61.238399, 1.838646)
  point P45 (56.238399, -1.860755)
  point P46 (56.238399, -7.259557)
  point P47 (61.238399, -10.958958)
  point P48 (61.238399, -5.560156)
  point P49 (56.238399, -9.259557)
  point P50 (53.822953, -9.933295)
  point P51 (51.513552, -9.933295)
  point P52 (47.212217, -9.933295)
  point P53 (46.646153, -14.965075)
  point P54 (52.072793, -14.953256)
  point P55 (44.902816, -9.933295)
  point P56 (41.007851, -9.933295)
  point P57 (38.69845, -9.933295)
  point P58 (34.397116, -9.933295)
  point P59 (33.814917, -14.99302)
  point P60 (39.273785, -14.981131)
  point P61 (21.918249, -17.914474)
  point P62 (26.474777, -15.009006)
  point P63 (32.087715, -9.933295)
  point P64 (28.19275, -9.933295)
  point P65 (61.238399, -12.958958)
  point P66 (59.477388, -14.93713)
  point P67 (-0.377778, 1.838646)
  point P68 (-1.595709, -3.560156)
  point P69 (-1.422914, -2.038404)
  point P70 (52.668252, -9.933295)
  point P71 (53.226043, -14.950744)
  point P72 (61.238399, 2.838646)
  point P73 (58.46709, 5.566705)
  point P74 (53.073781, 5.566705)
  point P75 (52.810441, 0.566705)
  point P76 (28.586061, -0.860755)
  point P77 (32.477893, -0.511209)
  point P78 (40.617673, -0.511209)
  point P79 (45.292994, -0.511209)
  point P80 (4.403231, 7.538047)
  point P81 (6.998769, 9.14927)
  point P82 (26.243893, 5.488791)
  point P83 (20.179892, -18.90355)
  point P84 (27.443577, 5.566705)
  point P85 (27.398593, 5.488791)
  point P86 (21.777262, 8.549964)
  point P87 (-1.643334, -5.560156)
  point P88 (-3.044173, -5.560156)
  point P89 (-1.858559, -10.958958)
  point P90 (-0.370905, -10.958958)
  point P91 (13.488058, -20.110558)
  point P92 (9.13463, -19.357761)
  point P93 (28.334938, 0.566705)
  point P94 (31.945526, 0.566705)
  point P95 (2.651998, 8.056851)
  point P96 (7.213176, 10.954264)
  dimension "d197" = 6.234
  dimension "d198" = 1
  dimension "d202" = 1.5
  dimension "d205" = 1.5
  dimension "d206" = 1.5
  dimension "d209" = 1
  dimension "d210" = 1
  dimension "d211" = 1
  dimension "d212" = 1
  constraints: 912 end point, 352 symmetric about line, 8 point on circle, 6 coincident, 5 parallel, 4 centre point, 3 horizontal, 3 perpendicular, 1 collinear, 1 point on line, 1 tangent, 1 vertical, 36 other
  measures "d197" distance of L0.start L2.end
  measures "d198" distance between parallel lines of L9 L3
  measures "d202" distance between parallel lines of L249 L245
  measures "d209" distance between parallel lines of L279 L289
  measures "d210" distance between parallel lines of L286 L285
  measures "d211" distance between parallel lines of L287 L283